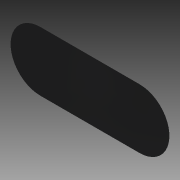
# Autodesk Inventor part: Trigger_Velostat
Saved by Autodesk Inventor 2014 SP1 (Build 180222100, 222)
## iProperties
Created: 2014-01-12
Part Number: Trigger_Velostat
Material: Rubber
Document SubType Name: Modeling
Designer: tuleu
Density: 0.93 g/cm^3
Appearance: Rubber - Black - Version 1.1
Author: tuleu
Autodesk Inventor part; units mm, degrees
ref_plane "YZ Plane" through (0, 0, 0) normal (1, 0, 0) x (0, 1, 0)
ref_plane "XZ Plane" through (0, 0, 0) normal (0, 1, 0) x (-1, 0, 0)
ref_plane "XY Plane" through (0, 0, 0) normal (0, 0, 1) x (1, 0, 0)
sketch "Sketch1" plane through (0, 0, 0) normal (0, 1, 0) x (-1, 0, 0)
  line L0 (75, -45) -> (-75, -45)
  line L1 (-75, 45) -> (75, 45)
  arc A0 (75, -45) -> (75, 45) centre (75, 0) ccw
  arc A1 (-75, 45) -> (-75, -45) centre (-75, 0) ccw
  line L2 (0, -45) -> (0, 45) construction
  line L3 (75, 0) -> (-75, 0) construction
  point P0 (0, 0)
  dimension "d1" = 45
  dimension "d2" = 150
  dimension "d3" = 90
  constraints: 8 end point, 4 midpoint, 4 point on circle, 2 centre point, 1 equal radius, 1 horizontal, 1 parallel, 1 perpendicular
  measures "d1" radius of A0
  measures "d2" distance of L3.start L3.end
  measures "d3" distance between parallel lines of L0 L1
extrude "Extrusion1" add sketch "Sketch1" along normal mid plane 0.01
body "Solid1"
